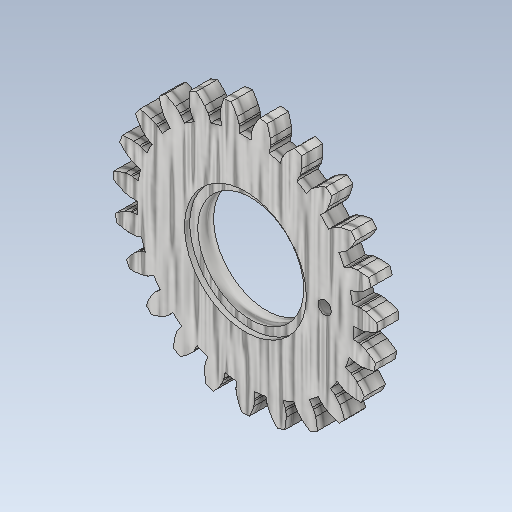
# Autodesk Inventor part: 横回転最終段
Saved by Autodesk Inventor 2020 (Build 240168000, 168)
## iProperties
Created: 2019-09-03
Part Number: 横回転最終段
Material: アルミニウム 7075
Document SubType Name: Modeling
Designer: tanjihayato
Density: 2.81 g/cm^3
Appearance: サテン - ブラシ仕上げ 重厚
Mass: 14.4164 g
Surface Area: 41.1785 cm^2
Volume: 5.1304 cm^3
Author: tanjihayato
Autodesk Inventor part; units mm, degrees
(part 1 of 2)
ref_plane "YZ Plane" through (0, 0, 0) normal (1, 0, 0) x (0, 1, 0)
ref_plane "XZ Plane" through (0, 0, 0) normal (0, 1, 0) x (-1, 0, 0)
ref_plane "XY Plane" through (0, 0, 0) normal (0, 0, 1) x (1, 0, 0)
sketch "スケッチ1" plane through (0, 0, 0) normal (0, 0, 1) x (1, 0, 0)
  arc A0 (24.5293, 43.4891) -> (24.4713, 43.1545) centre (26.6131, 42.9555) ccw
  arc A1 (24.8948, 44.5351) -> (24.5293, 43.4891) centre (30.276, 42.0681) ccw
  arc A2 (26.0165, 46.4263) -> (24.8948, 44.5351) centre (34.2234, 40.2803) ccw
  arc A3 (18.5713, 43.0032) -> (18.6058, 42.6653) centre (20.7218, 43.0516) ccw
  arc A4 (18.6411, 44.109) -> (18.5713, 43.0032) centre (24.4883, 43.1853) ccw
  arc A5 (19.2109, 46.2327) -> (18.6411, 44.109) centre (28.7717, 42.5289) ccw
  arc A6 (12.9654, 40.9279) -> (13.0897, 40.6118) centre (15.0231, 41.5547) ccw
  arc A7 (12.7342, 42.0115) -> (12.9654, 40.9279) centre (18.6138, 42.6996) ccw
  arc A8 (12.7099, 44.2101) -> (12.7342, 42.0115) centre (22.9154, 43.2231) ccw
  arc A9 (8.1272, 37.417) -> (8.3322, 37.1462) centre (9.9395, 38.5758) ccw
  arc A10 (7.6122, 38.3981) -> (8.1272, 37.417) centre (13.0882, 40.647) ccw
  arc A11 (6.9957, 40.5086) -> (7.6122, 38.3981) centre (17.089, 42.3117) ccw
  arc A12 (4.4157, 32.7311) -> (4.6861, 32.5256) centre (5.8481, 34.3358) ccw
  arc A13 (3.6551, 33.5368) -> (4.4157, 32.7311) centre (8.3213, 37.1797) ccw
  arc A14 (2.492, 35.4027) -> (3.6551, 33.5368) centre (11.7246, 39.8621) ccw
  arc A15 (2.106, 27.2175) -> (2.4219, 27.0926) centre (3.0524, 29.1491) ccw
  arc A16 (1.1563, 27.7881) -> (2.106, 27.2175) centre (4.6666, 32.5549) ccw
  arc A17 (-0.4671, 29.2711) -> (1.1563, 27.7881) centre (7.22, 36.056) ccw
  arc A18 (1.3696, 21.2852) -> (1.7074, 21.2502) centre (1.7597, 23.4006) ccw
  arc A19 (0.3011, 21.5785) -> (1.3696, 21.2852) centre (2.3951, 27.1155) ccw
  arc A20 (-1.6622, 22.5685) -> (0.3011, 21.5785) centre (3.9093, 31.1757) ccw
  arc A21 (2.2609, 15.3743) -> (2.5957, 15.4317) centre (2.0659, 17.5165) ccw
  arc A22 (1.153, 15.3684) -> (2.2609, 15.3743) centre (1.6755, 21.2651) ccw
  arc A23 (-1.0046, 15.792) -> (1.153, 15.3684) centre (2.0381, 25.5832) ccw
  arc A24 (4.714, 9.923) -> (5.0209, 10.0686) centre (3.9482, 11.9331) ccw
  arc A25 (3.6487, 9.6184) -> (4.714, 9.923) centre (2.5609, 15.4374) ccw
  arc A26 (1.4568, 9.4442) -> (3.6487, 9.6184) centre (1.7451, 19.6932) ccw
  arc A27 (8.5468, 5.3357) -> (8.803, 5.5587) centre (7.2671, 7.0647) ccw
  arc A28 (7.6032, 4.755) -> (8.5468, 5.3357) centre (4.9858, 10.0647) ccw
  arc A29 (5.5396, 3.9959) -> (7.6032, 4.755) centre (3.052, 13.9426) ccw
  arc A30 (13.4752, 1.9526) -> (13.6617, 2.2365) centre (11.7765, 3.2722) ccw
  arc A31 (12.7232, 1.1388) -> (13.4752, 1.9526) centre (8.7704, 5.5455) ccw
  arc A32 (10.941, -0.1489) -> (12.7232, 1.1388) centre (5.862, 8.7579) ccw
  arc A33 (19.1335, 0.0246) -> (19.2365, 0.3483) centre (17.1418, 0.837) ccw
  arc A34 (18.629, -0.9619) -> (19.1335, 0.0246) centre (13.6338, 2.2149) ccw
  arc A35 (17.2603, -2.6827) -> (18.629, -0.9619) centre (9.9666, 4.5235) ccw
  arc A36 (25.1022, -0.3053) -> (25.1141, 0.0342) centre (22.9651, -0.0604) ccw
  arc A37 (24.8825, -1.3913) -> (25.1022, -0.3053) centre (19.2155, 0.32) ccw
  arc A38 (24.0288, -3.4176) -> (24.8825, -1.3913) centre (15.0614, 1.5536) ccw
  arc A39 (30.9385, 0.9874) -> (30.8584, 1.3174) centre (28.8146, 0.6466) ccw
  arc A40 (31.02, -0.1176) -> (30.9385, 0.9874) centre (25.1014, 0.0013) ccw
  arc A41 (30.7446, -2.2991) -> (31.02, -0.1176) centre (20.7686, 0.0683) ccw
  arc A42 (36.2097, 3.8067) -> (36.0435, 4.1029) centre (34.2565, 2.9056) ccw
  arc A43 (36.5863, 2.7647) -> (36.2097, 3.8067) centre (30.8551, 1.2824) ccw
  arc A44 (36.9097, 0.5898) -> (36.5863, 2.7647) centre (26.6648, 0.178) ccw
  arc A45 (40.5247, 7.9437) -> (40.2848, 8.184) centre (38.8871, 6.549) ccw
  arc A46 (41.1685, 7.0419) -> (40.5247, 7.9437) centre (36.0497, 4.0683) ccw
  arc A47 (42.0667, 5.0349) -> (41.1685, 7.0419) centre (32.3128, 1.8743) ccw
  arc A48 (43.5636, 13.0914) -> (43.2677, 13.2581) centre (42.363, 11.3066) ccw
  arc A49 (44.4268, 12.3967) -> (43.5636, 13.0914) centre (40.3002, 8.1524) ccw
  arc A50 (45.8331, 10.7065) -> (44.4268, 12.3967) centre (37.2938, 5.0316) ccw
  arc A51 (45.101, 18.8681) -> (44.7711, 18.9488) centre (44.4264, 16.8256) ccw
  arc A52 (46.1196, 18.4321) -> (45.101, 18.8681) centre (43.2911, 13.2318) ccw
  arc A53 (47.9298, 17.184) -> (46.1196, 18.4321) centre (41.2381, 9.4156) ccw
  arc A54 (45.0228, 24.8454) -> (44.6833, 24.8341) centre (44.9243, 22.6966) ccw
  arc A55 (46.1213, 24.7004) -> (45.0228, 24.8454) centre (44.8007, 18.9297) ccw
  arc A56 (48.2011, 23.9869) -> (46.1213, 24.7004) centre (43.8535, 14.7012) ccw
  arc A57 (43.3349, 30.5799) -> (43.011, 30.4774) centre (43.8198, 28.4842) ccw
  arc A58 (44.4317, 30.7366) -> (43.3349, 30.5799) centre (44.717, 24.8237) ccw
  arc A59 (46.6269, 30.6108) -> (44.4317, 30.7366) centre (44.9458, 20.4964) ccw
  arc A60 (40.1624, 35.6464) -> (39.8782, 35.4603) centre (41.1947, 33.7593) ccw
  arc A61 (41.1763, 36.0932) -> (40.1624, 35.6464) centre (43.0462, 30.4765) ccw
  arc A62 (43.324, 36.5643) -> (41.1763, 36.0932) centre (44.434, 26.3714) ccw
  arc A63 (35.7406, 39.669) -> (35.5172, 39.4132) centre (37.2438, 38.1304) ccw
  arc A64 (36.5963, 40.3728) -> (35.7406, 39.669) centre (39.9123, 35.469) ccw
  arc A65 (38.5373, 41.4059) -> (36.5963, 40.3728) centre (42.3562, 31.8905) ccw
  arc A66 (30.3975, 42.3495) -> (30.2514, 42.043) centre (32.2601, 41.2736) ccw
  arc A67 (31.0316, 43.2581) -> (30.3975, 42.3495) centre (35.5477, 39.4308) ccw
  arc A68 (32.6219, 44.7765) -> (31.0316, 43.2581) centre (38.8664, 36.6443) ccw
  arc A69 (22.1646, 43.1545) -> (22.1065, 43.4891) centre (20.0227, 42.9555) ccw
  arc A70 (22.1065, 43.4891) -> (21.7411, 44.5351) centre (16.3598, 42.0681) ccw
  arc A71 (21.7411, 44.5351) -> (20.6194, 46.4263) centre (12.4124, 40.2803) ccw
  arc A72 (16.3845, 42.043) -> (16.2384, 42.3495) centre (14.3758, 41.2736) ccw
  arc A73 (16.2384, 42.3495) -> (15.6043, 43.2581) centre (11.0882, 39.4308) ccw
  arc A74 (15.6043, 43.2581) -> (14.014, 44.7765) centre (7.7695, 36.6443) ccw
  arc A75 (11.1187, 39.4132) -> (10.8953, 39.669) centre (9.3921, 38.1304) ccw
  arc A76 (10.8953, 39.669) -> (10.0396, 40.3728) centre (6.7235, 35.469) ccw
  arc A77 (10.0396, 40.3728) -> (8.0986, 41.4059) centre (4.2797, 31.8905) ccw
  arc A78 (6.7577, 35.4603) -> (6.4735, 35.6464) centre (5.4412, 33.7593) ccw
  arc A79 (6.4735, 35.6464) -> (5.4596, 36.0932) centre (3.5896, 30.4765) ccw
  arc A80 (5.4596, 36.0932) -> (3.3119, 36.5643) centre (2.2019, 26.3714) ccw
  arc A81 (3.6249, 30.4774) -> (3.301, 30.5799) centre (2.8161, 28.4842) ccw
  arc A82 (3.301, 30.5799) -> (2.2042, 30.7366) centre (1.9189, 24.8237) ccw
  arc A83 (2.2042, 30.7366) -> (0.009, 30.6108) centre (1.6901, 20.4964) ccw
  arc A84 (1.9526, 24.8341) -> (1.6131, 24.8454) centre (1.7116, 22.6966) ccw
  arc A85 (1.6131, 24.8454) -> (0.5146, 24.7004) centre (1.8352, 18.9297) ccw
  arc A86 (0.5146, 24.7004) -> (-1.5652, 23.9869) centre (2.7824, 14.7012) ccw
  arc A87 (1.8648, 18.9488) -> (1.5349, 18.8681) centre (2.2095, 16.8256) ccw
  arc A88 (1.5349, 18.8681) -> (0.5163, 18.4321) centre (3.3448, 13.2318) ccw
  arc A89 (0.5163, 18.4321) -> (-1.2939, 17.184) centre (5.3978, 9.4156) ccw
  arc A90 (3.3682, 13.2581) -> (3.0723, 13.0914) centre (4.2729, 11.3066) ccw
  arc A91 (3.0723, 13.0914) -> (2.2091, 12.3967) centre (6.3357, 8.1524) ccw
  arc A92 (2.2091, 12.3967) -> (0.8027, 10.7065) centre (9.3421, 5.0316) ccw
  arc A93 (6.3511, 8.184) -> (6.1112, 7.9437) centre (7.7488, 6.549) ccw
  arc A94 (6.1112, 7.9437) -> (5.4674, 7.0419) centre (10.5861, 4.0683) ccw
  arc A95 (5.4674, 7.0419) -> (4.5692, 5.0349) centre (14.323, 1.8743) ccw
  arc A96 (10.5924, 4.1029) -> (10.4262, 3.8067) centre (12.3794, 2.9056) ccw
  arc A97 (10.4262, 3.8067) -> (10.0496, 2.7647) centre (15.7808, 1.2824) ccw
  arc A98 (10.0496, 2.7647) -> (9.7262, 0.5898) centre (19.9711, 0.178) ccw
  arc A99 (15.7775, 1.3174) -> (15.6974, 0.9874) centre (17.8212, 0.6466) ccw
  arc A100 (15.6974, 0.9874) -> (15.6159, -0.1176) centre (21.5345, 0.0013) ccw
  arc A101 (15.6159, -0.1176) -> (15.8912, -2.2991) centre (25.8673, 0.0683) ccw
  arc A102 (21.5218, 0.0342) -> (21.5337, -0.3053) centre (23.6708, -0.0604) ccw
  arc A103 (21.5337, -0.3053) -> (21.7534, -1.3913) centre (27.4204, 0.32) ccw
  arc A104 (21.7534, -1.3913) -> (22.6071, -3.4176) centre (31.5745, 1.5536) ccw
  arc A105 (27.3994, 0.3483) -> (27.5024, 0.0246) centre (29.4941, 0.837) ccw
  arc A106 (27.5024, 0.0246) -> (28.0069, -0.9619) centre (33.0021, 2.2149) ccw
  arc A107 (28.0069, -0.9619) -> (29.3756, -2.6827) centre (36.6693, 4.5235) ccw
  arc A108 (32.9742, 2.2365) -> (33.1607, 1.9526) centre (34.8594, 3.2722) ccw
  arc A109 (33.1607, 1.9526) -> (33.9127, 1.1388) centre (37.8655, 5.5455) ccw
  arc A110 (33.9127, 1.1388) -> (35.6949, -0.1489) centre (40.7739, 8.7579) ccw
  arc A111 (37.8329, 5.5587) -> (38.0891, 5.3357) centre (39.3688, 7.0647) ccw
  arc A112 (38.0891, 5.3357) -> (39.0327, 4.755) centre (41.65, 10.0647) ccw
  arc A113 (39.0327, 4.755) -> (41.0963, 3.9959) centre (43.5839, 13.9426) ccw
  arc A114 (41.615, 10.0686) -> (41.9219, 9.923) centre (42.6877, 11.9331) ccw
  arc A115 (41.9219, 9.923) -> (42.9872, 9.6184) centre (44.0749, 15.4374) ccw
  arc A116 (42.9872, 9.6184) -> (45.1791, 9.4442) centre (44.8908, 19.6932) ccw
  arc A117 (44.0402, 15.4317) -> (44.3749, 15.3743) centre (44.57, 17.5165) ccw
  arc A118 (44.3749, 15.3743) -> (45.4829, 15.3684) centre (44.9604, 21.2651) ccw
  arc A119 (45.4829, 15.3684) -> (47.6405, 15.792) centre (44.5978, 25.5832) ccw
  arc A120 (44.9285, 21.2502) -> (45.2663, 21.2852) centre (44.8762, 23.4006) ccw
  arc A121 (45.2663, 21.2852) -> (46.3348, 21.5785) centre (44.2407, 27.1155) ccw
  arc A122 (46.3348, 21.5785) -> (48.2981, 22.5685) centre (42.7266, 31.1757) ccw
  arc A123 (44.214, 27.0926) -> (44.5299, 27.2175) centre (43.5835, 29.1491) ccw
  arc A124 (44.5299, 27.2175) -> (45.4796, 27.7881) centre (41.9693, 32.5549) ccw
  arc A125 (45.4796, 27.7881) -> (47.103, 29.2711) centre (39.4159, 36.056) ccw
  arc A126 (41.9498, 32.5256) -> (42.2202, 32.7311) centre (40.7878, 34.3358) ccw
  arc A127 (42.2202, 32.7311) -> (42.9808, 33.5368) centre (38.3146, 37.1797) ccw
  arc A128 (42.9808, 33.5368) -> (44.1439, 35.4027) centre (34.9113, 39.8621) ccw
  arc A129 (38.3037, 37.1462) -> (38.5087, 37.417) centre (36.6964, 38.5758) ccw
  arc A130 (38.5087, 37.417) -> (39.0237, 38.3981) centre (33.5477, 40.647) ccw
  arc A131 (39.0237, 38.3981) -> (39.6402, 40.5086) centre (29.5469, 42.3117) ccw
  arc A132 (33.5462, 40.6118) -> (33.6705, 40.9279) centre (31.6128, 41.5547) ccw
  arc A133 (33.6705, 40.9279) -> (33.9017, 42.0115) centre (28.0221, 42.6996) ccw
  arc A134 (33.9017, 42.0115) -> (33.926, 44.2101) centre (23.7205, 43.2231) ccw
  arc A135 (28.0301, 42.6653) -> (28.0645, 43.0032) centre (25.9141, 43.0516) ccw
  arc A136 (28.0645, 43.0032) -> (27.9948, 44.109) centre (22.1476, 43.1853) ccw
  arc A137 (27.9948, 44.109) -> (27.425, 46.2327) centre (17.8642, 42.5289) ccw
  arc A138 (24.4119, 42.0431) -> (22.2239, 42.0431) centre (23.3179, 21.5723) ccw
  arc A139 (18.8484, 41.5792) -> (16.7416, 40.9888) centre (23.3179, 21.5723) ccw
  arc A140 (13.6164, 39.6314) -> (11.7469, 38.4945) centre (23.3179, 21.5723) ccw
  arc A141 (9.1039, 36.3443) -> (7.6104, 34.7452) centre (23.3179, 21.5723) ccw
  arc A142 (5.6455, 31.9616) -> (4.6389, 30.0189) centre (23.3179, 21.5723) ccw
  arc A143 (3.4979, 26.8083) -> (3.0527, 24.6661) centre (23.3179, 21.5723) ccw
  arc A144 (2.8202, 21.2668) -> (2.9695, 19.0839) centre (23.3179, 21.5723) ccw
  arc A145 (3.6628, 15.7479) -> (4.3955, 13.6862) centre (23.3179, 21.5723) ccw
  arc A146 (5.963, 10.661) -> (7.2248, 8.8735) centre (23.3179, 21.5723) ccw
  arc A147 (9.5505, 6.3833) -> (11.2477, 5.0025) centre (23.3179, 21.5723) ccw
  arc A148 (14.1589, 3.2321) -> (16.1658, 2.3604) centre (23.3179, 21.5723) ccw
  arc A149 (19.4467, 1.4412) -> (21.6143, 1.1432) centre (23.3179, 21.5723) ccw
  arc A150 (25.0216, 1.1432) -> (27.1892, 1.4412) centre (23.3179, 21.5723) ccw
  arc A151 (30.4701, 2.3604) -> (32.477, 3.2321) centre (23.3179, 21.5723) ccw
  arc A152 (35.3882, 5.0025) -> (37.0854, 6.3833) centre (23.3179, 21.5723) ccw
  arc A153 (39.4111, 8.8735) -> (40.6728, 10.661) centre (23.3179, 21.5723) ccw
  arc A154 (42.2404, 13.6862) -> (42.9731, 15.7479) centre (23.3179, 21.5723) ccw
  arc A155 (43.6664, 19.0839) -> (43.8157, 21.2668) centre (23.3179, 21.5723) ccw
  arc A156 (43.5831, 24.6661) -> (43.138, 26.8083) centre (23.3179, 21.5723) ccw
  arc A157 (41.997, 30.0189) -> (40.9903, 31.9616) centre (23.3179, 21.5723) ccw
  arc A158 (39.0254, 34.7452) -> (37.532, 36.3443) centre (23.3179, 21.5723) ccw
  arc A159 (34.889, 38.4945) -> (33.0195, 39.6314) centre (23.3179, 21.5723) ccw
  arc A160 (29.8943, 40.9888) -> (27.7875, 41.5792) centre (23.3179, 21.5723) ccw
  arc A161 (20.6194, 46.4263) -> (19.2109, 46.2327) centre (23.3179, 21.5723) ccw
  arc A162 (14.014, 44.7765) -> (12.7099, 44.2101) centre (23.3179, 21.5723) ccw
  arc A163 (8.0986, 41.4059) -> (6.9957, 40.5086) centre (23.3179, 21.5723) ccw
  arc A164 (3.3119, 36.5643) -> (2.492, 35.4027) centre (23.3179, 21.5723) ccw
  arc A165 (0.009, 30.6108) -> (-0.4671, 29.2711) centre (23.3179, 21.5723) ccw
  arc A166 (-1.5652, 23.9869) -> (-1.6622, 22.5685) centre (23.3179, 21.5723) ccw
  arc A167 (-1.2939, 17.184) -> (-1.0046, 15.792) centre (23.3179, 21.5723) ccw
  arc A168 (0.8027, 10.7065) -> (1.4568, 9.4442) centre (23.3179, 21.5723) ccw
  arc A169 (4.5692, 5.0349) -> (5.5396, 3.9959) centre (23.3179, 21.5723) ccw
  arc A170 (9.7262, 0.5898) -> (10.941, -0.1489) centre (23.3179, 21.5723) ccw
  arc A171 (15.8912, -2.2991) -> (17.2603, -2.6827) centre (23.3179, 21.5723) ccw
  arc A172 (22.6071, -3.4176) -> (24.0288, -3.4176) centre (23.3179, 21.5723) ccw
  arc A173 (29.3756, -2.6827) -> (30.7446, -2.2991) centre (23.3179, 21.5723) ccw
  arc A174 (35.6949, -0.1489) -> (36.9097, 0.5898) centre (23.3179, 21.5723) ccw
  arc A175 (41.0963, 3.9959) -> (42.0667, 5.0349) centre (23.3179, 21.5723) ccw
  arc A176 (45.1791, 9.4442) -> (45.8331, 10.7065) centre (23.3179, 21.5723) ccw
  arc A177 (47.6405, 15.792) -> (47.9298, 17.184) centre (23.3179, 21.5723) ccw
  arc A178 (48.2981, 22.5685) -> (48.2011, 23.9869) centre (23.3179, 21.5723) ccw
  arc A179 (47.103, 29.2711) -> (46.6269, 30.6108) centre (23.3179, 21.5723) ccw
  arc A180 (44.1439, 35.4027) -> (43.324, 36.5643) centre (23.3179, 21.5723) ccw
  arc A181 (39.6402, 40.5086) -> (38.5373, 41.4059) centre (23.3179, 21.5723) ccw
  arc A182 (33.926, 44.2101) -> (32.6219, 44.7765) centre (23.3179, 21.5723) ccw
  arc A183 (27.425, 46.2327) -> (26.0165, 46.4263) centre (23.3179, 21.5723) ccw
  line L0 (24.4119, 42.0431) -> (24.4713, 43.1545)
  line L1 (18.8484, 41.5792) -> (18.6058, 42.6653)
  line L2 (13.6164, 39.6314) -> (13.0897, 40.6118)
  line L3 (9.1039, 36.3443) -> (8.3322, 37.1462)
  line L4 (5.6455, 31.9616) -> (4.6861, 32.5256)
  line L5 (3.4979, 26.8083) -> (2.4219, 27.0926)
  line L6 (2.8202, 21.2668) -> (1.7074, 21.2502)
  line L7 (3.6628, 15.7479) -> (2.5957, 15.4317)
  line L8 (5.963, 10.661) -> (5.0209, 10.0686)
  line L9 (9.5505, 6.3833) -> (8.803, 5.5587)
  line L10 (14.1589, 3.2321) -> (13.6617, 2.2365)
  line L11 (19.4467, 1.4412) -> (19.2365, 0.3483)
  line L12 (25.0216, 1.1432) -> (25.1141, 0.0342)
  line L13 (30.4701, 2.3604) -> (30.8584, 1.3174)
  line L14 (35.3882, 5.0025) -> (36.0435, 4.1029)
  line L15 (39.4111, 8.8735) -> (40.2848, 8.184)
  line L16 (42.2404, 13.6862) -> (43.2677, 13.2581)
  line L17 (43.6664, 19.0839) -> (44.7711, 18.9488)
  line L18 (43.5831, 24.6661) -> (44.6833, 24.8341)
  line L19 (41.997, 30.0189) -> (43.011, 30.4774)
  line L20 (39.0254, 34.7452) -> (39.8782, 35.4603)
  line L21 (34.889, 38.4945) -> (35.5172, 39.4132)
  line L22 (29.8943, 40.9888) -> (30.2514, 42.043)
  line L23 (22.2239, 42.0431) -> (22.1646, 43.1545)
  line L24 (16.7416, 40.9888) -> (16.3845, 42.043)
  line L25 (11.7469, 38.4945) -> (11.1187, 39.4132)
  line L26 (7.6104, 34.7452) -> (6.7577, 35.4603)
  line L27 (4.6389, 30.0189) -> (3.6249, 30.4774)
  line L28 (3.0527, 24.6661) -> (1.9526, 24.8341)
  line L29 (2.9695, 19.0839) -> (1.8648, 18.9488)
  line L30 (4.3955, 13.6862) -> (3.3682, 13.2581)
  line L31 (7.2248, 8.8735) -> (6.3511, 8.184)
  line L32 (11.2477, 5.0025) -> (10.5924, 4.1029)
  line L33 (16.1658, 2.3604) -> (15.7775, 1.3174)
  line L34 (21.6143, 1.1432) -> (21.5218, 0.0342)
  line L35 (27.1892, 1.4412) -> (27.3994, 0.3483)
  line L36 (32.477, 3.2321) -> (32.9742, 2.2365)
  line L37 (37.0854, 6.3833) -> (37.8329, 5.5587)
  line L38 (40.6728, 10.661) -> (41.615, 10.0686)
  line L39 (42.9731, 15.7479) -> (44.0402, 15.4317)
  line L40 (43.8157, 21.2668) -> (44.9285, 21.2502)
  line L41 (43.138, 26.8083) -> (44.214, 27.0926)
  line L42 (40.9903, 31.9616) -> (41.9498, 32.5256)
  line L43 (37.532, 36.3443) -> (38.3037, 37.1462)
  line L44 (33.0195, 39.6314) -> (33.5462, 40.6118)
  line L45 (27.7875, 41.5792) -> (28.0301, 42.6653)
  line L46 (-3.6821, 21.5723) -> (50.3179, 21.5723)
  line L47 (23.3179, -5.4277) -> (23.3179, 48.5723)
  point P0 (0, 0)
  point P1 (0, 0)
  constraints: 276 point on circle, 138 centre point, 96 end point, 2 horizontal alignment, 136 other
extrude "押し出し1" add sketch "スケッチ1" along normal blind 4
sketch "スケッチ2" plane through (0, 0, 4) normal (0, 0, 1) x (1, 0, 0)
  arc A0 (24.5293, 43.4891) -> (24.4713, 43.1545) centre (26.6131, 42.9555) ccw projected
  line L0 (24.4713, 43.1545) -> (24.4119, 42.0431) projected
  arc A1 (24.4119, 42.0431) -> (22.2239, 42.0431) centre (23.3179, 21.5723) ccw projected
  line L1 (22.2239, 42.0431) -> (22.1646, 43.1545) projected
  arc A2 (22.1646, 43.1545) -> (22.1065, 43.4891) centre (20.0227, 42.9555) ccw projected
  arc A3 (22.1065, 43.4891) -> (21.7411, 44.5351) centre (16.3598, 42.0681) ccw projected
  arc A4 (21.7411, 44.5351) -> (20.6194, 46.4263) centre (12.4124, 40.2803) ccw projected
  arc A5 (20.6194, 46.4263) -> (19.2109, 46.2327) centre (23.3179, 21.5723) ccw projected
  arc A6 (19.2109, 46.2327) -> (18.6411, 44.109) centre (28.7717, 42.5289) ccw projected
  arc A7 (18.6411, 44.109) -> (18.5713, 43.0032) centre (24.4883, 43.1853) ccw projected
  arc A8 (18.5713, 43.0032) -> (18.6058, 42.6653) centre (20.7218, 43.0516) ccw projected
  line L2 (18.6058, 42.6653) -> (18.8484, 41.5792) projected
  arc A9 (18.8484, 41.5792) -> (16.7416, 40.9888) centre (23.3179, 21.5723) ccw projected
  line L3 (16.7416, 40.9888) -> (16.3845, 42.043) projected
  arc A10 (16.3845, 42.043) -> (16.2384, 42.3495) centre (14.3758, 41.2736) ccw projected
  arc A11 (16.2384, 42.3495) -> (15.6043, 43.2581) centre (11.0882, 39.4308) ccw projected
  arc A12 (15.6043, 43.2581) -> (14.014, 44.7765) centre (7.7695, 36.6443) ccw projected
  arc A13 (14.014, 44.7765) -> (12.7099, 44.2101) centre (23.3179, 21.5723) ccw projected
  arc A14 (12.7099, 44.2101) -> (12.7342, 42.0115) centre (22.9154, 43.2231) ccw projected
  arc A15 (12.7342, 42.0115) -> (12.9654, 40.9279) centre (18.6138, 42.6996) ccw projected
  arc A16 (12.9654, 40.9279) -> (13.0897, 40.6118) centre (15.0231, 41.5547) ccw projected
  line L4 (13.0897, 40.6118) -> (13.6164, 39.6314) projected
  arc A17 (13.6164, 39.6314) -> (11.7469, 38.4945) centre (23.3179, 21.5723) ccw projected
  line L5 (11.7469, 38.4945) -> (11.1187, 39.4132) projected
  arc A18 (11.1187, 39.4132) -> (10.8953, 39.669) centre (9.3921, 38.1304) ccw projected
  arc A19 (10.8953, 39.669) -> (10.0396, 40.3728) centre (6.7235, 35.469) ccw projected
  arc A20 (10.0396, 40.3728) -> (8.0986, 41.4059) centre (4.2797, 31.8905) ccw projected
  arc A21 (8.0986, 41.4059) -> (6.9957, 40.5086) centre (23.3179, 21.5723) ccw projected
  arc A22 (6.9957, 40.5086) -> (7.6122, 38.3981) centre (17.089, 42.3117) ccw projected
  arc A23 (7.6122, 38.3981) -> (8.1272, 37.417) centre (13.0882, 40.647) ccw projected
  arc A24 (8.1272, 37.417) -> (8.3322, 37.1462) centre (9.9395, 38.5758) ccw projected
  line L6 (8.3322, 37.1462) -> (9.1039, 36.3443) projected
  arc A25 (9.1039, 36.3443) -> (7.6104, 34.7452) centre (23.3179, 21.5723) ccw projected
  line L7 (7.6104, 34.7452) -> (6.7577, 35.4603) projected
  arc A26 (6.7577, 35.4603) -> (6.4735, 35.6464) centre (5.4412, 33.7593) ccw projected
  arc A27 (6.4735, 35.6464) -> (5.4596, 36.0932) centre (3.5896, 30.4765) ccw projected
  arc A28 (5.4596, 36.0932) -> (3.3119, 36.5643) centre (2.2019, 26.3714) ccw projected
  arc A29 (3.3119, 36.5643) -> (2.492, 35.4027) centre (23.3179, 21.5723) ccw projected
  arc A30 (2.492, 35.4027) -> (3.6551, 33.5368) centre (11.7246, 39.8621) ccw projected
  arc A31 (3.6551, 33.5368) -> (4.4157, 32.7311) centre (8.3213, 37.1797) ccw projected
  arc A32 (4.4157, 32.7311) -> (4.6861, 32.5256) centre (5.8481, 34.3358) ccw projected
  line L8 (4.6861, 32.5256) -> (5.6455, 31.9616) projected
  arc A33 (5.6455, 31.9616) -> (4.6389, 30.0189) centre (23.3179, 21.5723) ccw projected
  line L9 (4.6389, 30.0189) -> (3.6249, 30.4774) projected
  arc A34 (3.6249, 30.4774) -> (3.301, 30.5799) centre (2.8161, 28.4842) ccw projected
  arc A35 (3.301, 30.5799) -> (2.2042, 30.7366) centre (1.9189, 24.8237) ccw projected
  arc A36 (2.2042, 30.7366) -> (0.009, 30.6108) centre (1.6901, 20.4964) ccw projected
  arc A37 (0.009, 30.6108) -> (-0.4671, 29.2711) centre (23.3179, 21.5723) ccw projected
  arc A38 (-0.4671, 29.2711) -> (1.1563, 27.7881) centre (7.22, 36.056) ccw projected
  arc A39 (1.1563, 27.7881) -> (2.106, 27.2175) centre (4.6666, 32.5549) ccw projected
  arc A40 (2.106, 27.2175) -> (2.4219, 27.0926) centre (3.0524, 29.1491) ccw projected
  line L10 (2.4219, 27.0926) -> (3.4979, 26.8083) projected
  arc A41 (3.4979, 26.8083) -> (3.0527, 24.6661) centre (23.3179, 21.5723) ccw projected
  line L11 (3.0527, 24.6661) -> (1.9526, 24.8341) projected
  arc A42 (1.9526, 24.8341) -> (1.6131, 24.8454) centre (1.7116, 22.6966) ccw projected
  arc A43 (1.6131, 24.8454) -> (0.5146, 24.7004) centre (1.8352, 18.9297) ccw projected
  arc A44 (0.5146, 24.7004) -> (-1.5652, 23.9869) centre (2.7824, 14.7012) ccw projected
  arc A45 (-1.5652, 23.9869) -> (-1.6622, 22.5685) centre (23.3179, 21.5723) ccw projected
  arc A46 (-1.6622, 22.5685) -> (0.3011, 21.5785) centre (3.9093, 31.1757) ccw projected
  arc A47 (0.3011, 21.5785) -> (1.3696, 21.2852) centre (2.3951, 27.1155) ccw projected
  arc A48 (1.3696, 21.2852) -> (1.7074, 21.2502) centre (1.7597, 23.4006) ccw projected
  line L12 (1.7074, 21.2502) -> (2.8202, 21.2668) projected
  arc A49 (2.8202, 21.2668) -> (2.9695, 19.0839) centre (23.3179, 21.5723) ccw projected
  line L13 (2.9695, 19.0839) -> (1.8648, 18.9488) projected
  arc A50 (1.8648, 18.9488) -> (1.5349, 18.8681) centre (2.2095, 16.8256) ccw projected
  arc A51 (1.5349, 18.8681) -> (0.5163, 18.4321) centre (3.3448, 13.2318) ccw projected
  arc A52 (0.5163, 18.4321) -> (-1.2939, 17.184) centre (5.3978, 9.4156) ccw projected
  arc A53 (-1.2939, 17.184) -> (-1.0046, 15.792) centre (23.3179, 21.5723) ccw projected
  arc A54 (-1.0046, 15.792) -> (1.153, 15.3684) centre (2.0381, 25.5832) ccw projected
  arc A55 (1.153, 15.3684) -> (2.2609, 15.3743) centre (1.6755, 21.2651) ccw projected
  arc A56 (2.2609, 15.3743) -> (2.5957, 15.4317) centre (2.0659, 17.5165) ccw projected
  line L14 (2.5957, 15.4317) -> (3.6628, 15.7479) projected
  arc A57 (3.6628, 15.7479) -> (4.3955, 13.6862) centre (23.3179, 21.5723) ccw projected
  line L15 (4.3955, 13.6862) -> (3.3682, 13.2581) projected
  arc A58 (3.3682, 13.2581) -> (3.0723, 13.0914) centre (4.2729, 11.3066) ccw projected
  arc A59 (3.0723, 13.0914) -> (2.2091, 12.3967) centre (6.3357, 8.1524) ccw projected
  arc A60 (2.2091, 12.3967) -> (0.8027, 10.7065) centre (9.3421, 5.0316) ccw projected
  arc A61 (0.8027, 10.7065) -> (1.4568, 9.4442) centre (23.3179, 21.5723) ccw projected
  arc A62 (1.4568, 9.4442) -> (3.6487, 9.6184) centre (1.7451, 19.6932) ccw projected
  arc A63 (3.6487, 9.6184) -> (4.714, 9.923) centre (2.5609, 15.4374) ccw projected
  arc A64 (4.714, 9.923) -> (5.0209, 10.0686) centre (3.9482, 11.9331) ccw projected
  line L16 (5.0209, 10.0686) -> (5.963, 10.661) projected
  arc A65 (5.963, 10.661) -> (7.2248, 8.8735) centre (23.3179, 21.5723) ccw projected
  line L17 (7.2248, 8.8735) -> (6.3511, 8.184) projected
  arc A66 (6.3511, 8.184) -> (6.1112, 7.9437) centre (7.7488, 6.549) ccw projected
  arc A67 (6.1112, 7.9437) -> (5.4674, 7.0419) centre (10.5861, 4.0683) ccw projected
  arc A68 (5.4674, 7.0419) -> (4.5692, 5.0349) centre (14.323, 1.8743) ccw projected
  arc A69 (4.5692, 5.0349) -> (5.5396, 3.9959) centre (23.3179, 21.5723) ccw projected
  arc A70 (5.5396, 3.9959) -> (7.6032, 4.755) centre (3.052, 13.9426) ccw projected
  arc A71 (7.6032, 4.755) -> (8.5468, 5.3357) centre (4.9858, 10.0647) ccw projected
  arc A72 (8.5468, 5.3357) -> (8.803, 5.5587) centre (7.2671, 7.0647) ccw projected
  line L18 (8.803, 5.5587) -> (9.5505, 6.3833) projected
  arc A73 (9.5505, 6.3833) -> (11.2477, 5.0025) centre (23.3179, 21.5723) ccw projected
  line L19 (11.2477, 5.0025) -> (10.5924, 4.1029) projected
  arc A74 (10.5924, 4.1029) -> (10.4262, 3.8067) centre (12.3794, 2.9056) ccw projected
  arc A75 (10.4262, 3.8067) -> (10.0496, 2.7647) centre (15.7808, 1.2824) ccw projected
  arc A76 (10.0496, 2.7647) -> (9.7262, 0.5898) centre (19.9711, 0.178) ccw projected
  arc A77 (9.7262, 0.5898) -> (10.941, -0.1489) centre (23.3179, 21.5723) ccw projected
  arc A78 (10.941, -0.1489) -> (12.7232, 1.1388) centre (5.862, 8.7579) ccw projected
  arc A79 (12.7232, 1.1388) -> (13.4752, 1.9526) centre (8.7704, 5.5455) ccw projected
  arc A80 (13.4752, 1.9526) -> (13.6617, 2.2365) centre (11.7765, 3.2722) ccw projected
  line L20 (13.6617, 2.2365) -> (14.1589, 3.2321) projected
  arc A81 (14.1589, 3.2321) -> (16.1658, 2.3604) centre (23.3179, 21.5723) ccw projected
  line L21 (16.1658, 2.3604) -> (15.7775, 1.3174) projected
  arc A82 (15.7775, 1.3174) -> (15.6974, 0.9874) centre (17.8212, 0.6466) ccw projected
  arc A83 (15.6974, 0.9874) -> (15.6159, -0.1176) centre (21.5345, 0.0013) ccw projected
  arc A84 (15.6159, -0.1176) -> (15.8912, -2.2991) centre (25.8673, 0.0683) ccw projected
  arc A85 (15.8912, -2.2991) -> (17.2603, -2.6827) centre (23.3179, 21.5723) ccw projected
  arc A86 (17.2603, -2.6827) -> (18.629, -0.9619) centre (9.9666, 4.5235) ccw projected
  arc A87 (18.629, -0.9619) -> (19.1335, 0.0246) centre (13.6338, 2.2149) ccw projected
  arc A88 (19.1335, 0.0246) -> (19.2365, 0.3483) centre (17.1418, 0.837) ccw projected
  line L22 (19.2365, 0.3483) -> (19.4467, 1.4412) projected
  arc A89 (19.4467, 1.4412) -> (21.6143, 1.1432) centre (23.3179, 21.5723) ccw projected
  line L23 (21.6143, 1.1432) -> (21.5218, 0.0342) projected
  arc A90 (21.5218, 0.0342) -> (21.5337, -0.3053) centre (23.6708, -0.0604) ccw projected
  arc A91 (21.5337, -0.3053) -> (21.7534, -1.3913) centre (27.4204, 0.32) ccw projected
  arc A92 (21.7534, -1.3913) -> (22.6071, -3.4176) centre (31.5745, 1.5536) ccw projected
  arc A93 (22.6071, -3.4176) -> (24.0288, -3.4176) centre (23.3179, 21.5723) ccw projected
  arc A94 (24.0288, -3.4176) -> (24.8825, -1.3913) centre (15.0614, 1.5536) ccw projected
  arc A95 (24.8825, -1.3913) -> (25.1022, -0.3053) centre (19.2155, 0.32) ccw projected
  arc A96 (25.1022, -0.3053) -> (25.1141, 0.0342) centre (22.9651, -0.0604) ccw projected
  line L24 (25.1141, 0.0342) -> (25.0216, 1.1432) projected
  arc A97 (25.0216, 1.1432) -> (27.1892, 1.4412) centre (23.3179, 21.5723) ccw projected
  line L25 (27.1892, 1.4412) -> (27.3994, 0.3483) projected
  arc A98 (27.3994, 0.3483) -> (27.5024, 0.0246) centre (29.4941, 0.837) ccw projected
  arc A99 (27.5024, 0.0246) -> (28.0069, -0.9619) centre (33.0021, 2.2149) ccw projected
  arc A100 (28.0069, -0.9619) -> (29.3756, -2.6827) centre (36.6693, 4.5235) ccw projected
  arc A101 (29.3756, -2.6827) -> (30.7446, -2.2991) centre (23.3179, 21.5723) ccw projected
  arc A102 (30.7446, -2.2991) -> (31.02, -0.1176) centre (20.7686, 0.0683) ccw projected
  arc A103 (31.02, -0.1176) -> (30.9385, 0.9874) centre (25.1014, 0.0013) ccw projected
  arc A104 (30.9385, 0.9874) -> (30.8584, 1.3174) centre (28.8146, 0.6466) ccw projected
  line L26 (30.8584, 1.3174) -> (30.4701, 2.3604) projected
  arc A105 (30.4701, 2.3604) -> (32.477, 3.2321) centre (23.3179, 21.5723) ccw projected
  line L27 (32.477, 3.2321) -> (32.9742, 2.2365) projected
  arc A106 (32.9742, 2.2365) -> (33.1607, 1.9526) centre (34.8594, 3.2722) ccw projected
  arc A107 (33.1607, 1.9526) -> (33.9127, 1.1388) centre (37.8655, 5.5455) ccw projected
  arc A108 (33.9127, 1.1388) -> (35.6949, -0.1489) centre (40.7739, 8.7579) ccw projected
  arc A109 (35.6949, -0.1489) -> (36.9097, 0.5898) centre (23.3179, 21.5723) ccw projected
  arc A110 (36.9097, 0.5898) -> (36.5863, 2.7647) centre (26.6648, 0.178) ccw projected
  arc A111 (36.5863, 2.7647) -> (36.2097, 3.8067) centre (30.8551, 1.2824) ccw projected
  arc A112 (36.2097, 3.8067) -> (36.0435, 4.1029) centre (34.2565, 2.9056) ccw projected
  line L28 (36.0435, 4.1029) -> (35.3882, 5.0025) projected
  arc A113 (35.3882, 5.0025) -> (37.0854, 6.3833) centre (23.3179, 21.5723) ccw projected
  line L29 (37.0854, 6.3833) -> (37.8329, 5.5587) projected
  arc A114 (37.8329, 5.5587) -> (38.0891, 5.3357) centre (39.3688, 7.0647) ccw projected
  arc A115 (38.0891, 5.3357) -> (39.0327, 4.755) centre (41.65, 10.0647) ccw projected
  arc A116 (39.0327, 4.755) -> (41.0963, 3.9959) centre (43.5839, 13.9426) ccw projected
  arc A117 (41.0963, 3.9959) -> (42.0667, 5.0349) centre (23.3179, 21.5723) ccw projected
  arc A118 (42.0667, 5.0349) -> (41.1685, 7.0419) centre (32.3128, 1.8743) ccw projected
  arc A119 (41.1685, 7.0419) -> (40.5247, 7.9437) centre (36.0497, 4.0683) ccw projected
  arc A120 (40.5247, 7.9437) -> (40.2848, 8.184) centre (38.8871, 6.549) ccw projected
  line L30 (40.2848, 8.184) -> (39.4111, 8.8735) projected
  arc A121 (39.4111, 8.8735) -> (40.6728, 10.661) centre (23.3179, 21.5723) ccw projected
  line L31 (40.6728, 10.661) -> (41.615, 10.0686) projected
  arc A122 (41.615, 10.0686) -> (41.9219, 9.923) centre (42.6877, 11.9331) ccw projected
  arc A123 (41.9219, 9.923) -> (42.9872, 9.6184) centre (44.0749, 15.4374) ccw projected
  arc A124 (42.9872, 9.6184) -> (45.1791, 9.4442) centre (44.8908, 19.6932) ccw projected
  arc A125 (45.1791, 9.4442) -> (45.8331, 10.7065) centre (23.3179, 21.5723) ccw projected
  arc A126 (45.8331, 10.7065) -> (44.4268, 12.3967) centre (37.2938, 5.0316) ccw projected
  arc A127 (44.4268, 12.3967) -> (43.5636, 13.0914) centre (40.3002, 8.1524) ccw projected
  arc A128 (43.5636, 13.0914) -> (43.2677, 13.2581) centre (42.363, 11.3066) ccw projected
  line L32 (43.2677, 13.2581) -> (42.2404, 13.6862) projected
  arc A129 (42.2404, 13.6862) -> (42.9731, 15.7479) centre (23.3179, 21.5723) ccw projected
  line L33 (42.9731, 15.7479) -> (44.0402, 15.4317) projected
  arc A130 (44.0402, 15.4317) -> (44.3749, 15.3743) centre (44.57, 17.5165) ccw projected
  arc A131 (44.3749, 15.3743) -> (45.4829, 15.3684) centre (44.9604, 21.2651) ccw projected
  arc A132 (45.4829, 15.3684) -> (47.6405, 15.792) centre (44.5978, 25.5832) ccw projected
  arc A133 (47.6405, 15.792) -> (47.9298, 17.184) centre (23.3179, 21.5723) ccw projected
  arc A134 (47.9298, 17.184) -> (46.1196, 18.4321) centre (41.2381, 9.4156) ccw projected
  arc A135 (46.1196, 18.4321) -> (45.101, 18.8681) centre (43.2911, 13.2318) ccw projected
  arc A136 (45.101, 18.8681) -> (44.7711, 18.9488) centre (44.4264, 16.8256) ccw projected
  line L34 (44.7711, 18.9488) -> (43.6664, 19.0839) projected
  arc A137 (43.6664, 19.0839) -> (43.8157, 21.2668) centre (23.3179, 21.5723) ccw projected
  line L35 (43.8157, 21.2668) -> (44.9285, 21.2502) projected
  arc A138 (44.9285, 21.2502) -> (45.2663, 21.2852) centre (44.8762, 23.4006) ccw projected
  arc A139 (45.2663, 21.2852) -> (46.3348, 21.5785) centre (44.2407, 27.1155) ccw projected
  arc A140 (46.3348, 21.5785) -> (48.2981, 22.5685) centre (42.7266, 31.1757) ccw projected
  arc A141 (48.2981, 22.5685) -> (48.2011, 23.9869) centre (23.3179, 21.5723) ccw projected
  arc A142 (48.2011, 23.9869) -> (46.1213, 24.7004) centre (43.8535, 14.7012) ccw projected
  arc A143 (46.1213, 24.7004) -> (45.0228, 24.8454) centre (44.8007, 18.9297) ccw projected
  arc A144 (45.0228, 24.8454) -> (44.6833, 24.8341) centre (44.9243, 22.6966) ccw projected
  line L36 (44.6833, 24.8341) -> (43.5831, 24.6661) projected
  arc A145 (43.5831, 24.6661) -> (43.138, 26.8083) centre (23.3179, 21.5723) ccw projected
  line L37 (43.138, 26.8083) -> (44.214, 27.0926) projected
  arc A146 (44.214, 27.0926) -> (44.5299, 27.2175) centre (43.5835, 29.1491) ccw projected
  arc A147 (44.5299, 27.2175) -> (45.4796, 27.7881) centre (41.9693, 32.5549) ccw projected
  arc A148 (45.4796, 27.7881) -> (47.103, 29.2711) centre (39.4159, 36.056) ccw projected
  arc A149 (47.103, 29.2711) -> (46.6269, 30.6108) centre (23.3179, 21.5723) ccw projected
  arc A150 (46.6269, 30.6108) -> (44.4317, 30.7366) centre (44.9458, 20.4964) ccw projected
  arc A151 (44.4317, 30.7366) -> (43.3349, 30.5799) centre (44.717, 24.8237) ccw projected
  arc A152 (43.3349, 30.5799) -> (43.011, 30.4774) centre (43.8198, 28.4842) ccw projected
  line L38 (43.011, 30.4774) -> (41.997, 30.0189) projected
  arc A153 (41.997, 30.0189) -> (40.9903, 31.9616) centre (23.3179, 21.5723) ccw projected
  line L39 (40.9903, 31.9616) -> (41.9498, 32.5256) projected
  arc A154 (41.9498, 32.5256) -> (42.2202, 32.7311) centre (40.7878, 34.3358) ccw projected
  arc A155 (42.2202, 32.7311) -> (42.9808, 33.5368) centre (38.3146, 37.1797) ccw projected
  arc A156 (42.9808, 33.5368) -> (44.1439, 35.4027) centre (34.9113, 39.8621) ccw projected
  arc A157 (44.1439, 35.4027) -> (43.324, 36.5643) centre (23.3179, 21.5723) ccw projected
  arc A158 (43.324, 36.5643) -> (41.1763, 36.0932) centre (44.434, 26.3714) ccw projected
  arc A159 (41.1763, 36.0932) -> (40.1624, 35.6464) centre (43.0462, 30.4765) ccw projected
  arc A160 (40.1624, 35.6464) -> (39.8782, 35.4603) centre (41.1947, 33.7593) ccw projected
  line L40 (39.8782, 35.4603) -> (39.0254, 34.7452) projected
  arc A161 (39.0254, 34.7452) -> (37.532, 36.3443) centre (23.3179, 21.5723) ccw projected
  line L41 (37.532, 36.3443) -> (38.3037, 37.1462) projected
  arc A162 (38.3037, 37.1462) -> (38.5087, 37.417) centre (36.6964, 38.5758) ccw projected
  arc A163 (38.5087, 37.417) -> (39.0237, 38.3981) centre (33.5477, 40.647) ccw projected
  arc A164 (39.0237, 38.3981) -> (39.6402, 40.5086) centre (29.5469, 42.3117) ccw projected
  arc A165 (39.6402, 40.5086) -> (38.5373, 41.4059) centre (23.3179, 21.5723) ccw projected
  arc A166 (38.5373, 41.4059) -> (36.5963, 40.3728) centre (42.3562, 31.8905) ccw projected
  arc A167 (36.5963, 40.3728) -> (35.7406, 39.669) centre (39.9123, 35.469) ccw projected
  arc A168 (35.7406, 39.669) -> (35.5172, 39.4132) centre (37.2438, 38.1304) ccw projected
  line L42 (35.5172, 39.4132) -> (34.889, 38.4945) projected
  arc A169 (34.889, 38.4945) -> (33.0195, 39.6314) centre (23.3179, 21.5723) ccw projected
  line L43 (33.0195, 39.6314) -> (33.5462, 40.6118) projected
  arc A170 (33.5462, 40.6118) -> (33.6705, 40.9279) centre (31.6128, 41.5547) ccw projected
  arc A171 (33.6705, 40.9279) -> (33.9017, 42.0115) centre (28.0221, 42.6996) ccw projected
  arc A172 (33.9017, 42.0115) -> (33.926, 44.2101) centre (23.7205, 43.2231) ccw projected
  arc A173 (33.926, 44.2101) -> (32.6219, 44.7765) centre (23.3179, 21.5723) ccw projected
  arc A174 (32.6219, 44.7765) -> (31.0316, 43.2581) centre (38.8664, 36.6443) ccw projected
  arc A175 (31.0316, 43.2581) -> (30.3975, 42.3495) centre (35.5477, 39.4308) ccw projected
  arc A176 (30.3975, 42.3495) -> (30.2514, 42.043) centre (32.2601, 41.2736) ccw projected
  line L44 (30.2514, 42.043) -> (29.8943, 40.9888) projected
  arc A177 (29.8943, 40.9888) -> (27.7875, 41.5792) centre (23.3179, 21.5723) ccw projected
  line L45 (27.7875, 41.5792) -> (28.0301, 42.6653) projected
  arc A178 (28.0301, 42.6653) -> (28.0645, 43.0032) centre (25.9141, 43.0516) ccw projected
  arc A179 (28.0645, 43.0032) -> (27.9948, 44.109) centre (22.1476, 43.1853) ccw projected
  arc A180 (27.9948, 44.109) -> (27.425, 46.2327) centre (17.8642, 42.5289) ccw projected
  arc A181 (27.425, 46.2327) -> (26.0165, 46.4263) centre (23.3179, 21.5723) ccw projected
  arc A182 (26.0165, 46.4263) -> (24.8948, 44.5351) centre (34.2234, 40.2803) ccw projected
  arc A183 (24.8948, 44.5351) -> (24.5293, 43.4891) centre (30.276, 42.0681) ccw projected
  circle A184 centre (38.3179, 21.5723) radius 1.25
  line L46 (23.3179, 21.5723) -> (38.3179, 21.5723) construction
  circle A185 centre (23.3179, 21.5723) radius 10.025
  point P0 (0, 0)
  dimension "d2" = 2.5
  dimension "d3" = 15
  dimension "d4" = 20.05
  constraints: 2 centre point, 2 end point, 1 coincident, 1 horizontal
  measures "d2" diameter of A184
  measures "d3" distance of L46.start L46.end
  measures "d4" diameter of A185
extrude "押し出し2" cut sketch "スケッチ2" against normal blind 4 contours A184 | A185